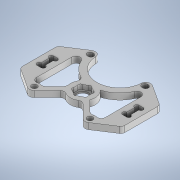
# Autodesk Inventor part: Leg_joint_roll_frame
Saved by Autodesk Inventor 2020 (Build 240168000, 168)
## iProperties
Created: 2021-10-17
Part Number: Leg_joint_roll_frame
Material: アルミニウム 2014-T4
Document SubType Name: Modeling
Designer: Masato Kubotera
Density: 2.8 g/cm^3
Appearance: 滑らか - 淡い灰色
Description: A2017 T3
Mass: 6.35026 g
Surface Area: 26.3941 cm^2
Volume: 2.26795 cm^3
Author: Masato Kubotera
Autodesk Inventor part; units mm, degrees
ref_plane "YZ Plane" through (0, 0, 0) normal (1, 0, 0) x (0, 1, 0)
ref_plane "XZ Plane" through (0, 0, 0) normal (0, 1, 0) x (-1, 0, 0)
ref_plane "XY Plane" through (0, 0, 0) normal (0, 0, 1) x (1, 0, 0)
derived "Leg_joint_roll_basis.ipt"
sketch "スケッチ1" plane through (0, 0, 0) normal (0, 0, 1) x (1, 0, 0)
  line L0 (0, 47.5) -> (0, -12.4) construction
  line L1 (-12.5, 47.5) -> (12.5, 47.5) construction
  line L2 (-12.5, 42.45) -> (-5.9323, -0.8988) construction
  arc A0 (-5.9323, -0.8988) -> (5.9323, -0.8988) centre (0, 0) ccw construction
  line L3 (-5.55, 45.05) -> (-3.45, 45.05) construction
  line L4 (5.55, 45.05) -> (5.55, 42.45) construction
  line L5 (5.55, 42.45) -> (3.45, 42.45) construction
  line L6 (-5.55, 42.45) -> (-5.55, 45.05) construction
  line L7 (-5.55, 45.05) -> (5.55, 42.45) construction
  line L8 (5.55, 45.05) -> (-5.55, 42.45) construction
  line L9 (-5.5, 45) -> (5.5, 45) construction
  line L10 (5.5, 45) -> (5.5, 42.5) construction
  line L11 (5.5, 42.5) -> (-5.5, 42.5) construction
  line L12 (-5.5, 42.5) -> (-5.5, 45) construction
  line L13 (-5.5, 45) -> (5.5, 42.5) construction
  line L14 (5.5, 45) -> (-5.5, 42.5) construction
  line L15 (-5.55, 43.75) -> (5.55, 43.75) construction
  arc A1 (-3.45, 45.05) -> (-5.55, 45.05) centre (-4.5, 45.05) ccw construction
  arc A2 (-5.55, 42.45) -> (-3.45, 42.45) centre (-4.5, 42.45) ccw construction
  line L16 (12.5, 42.45) -> (5.9323, -0.8988) construction
  arc A3 (5.55, 45.05) -> (3.45, 45.05) centre (4.5, 45.05) ccw construction
  arc A4 (3.45, 42.45) -> (5.55, 42.45) centre (4.5, 42.45) ccw construction
  line L17 (-3.45, 45.05) -> (3.45, 45.05) construction
  line L18 (-3.45, 42.45) -> (-5.55, 42.45) construction
  line L19 (3.45, 42.45) -> (-3.45, 42.45) construction
  line L20 (3.45, 45.05) -> (5.55, 45.05) construction
  circle A5 centre (0, 0) radius 4.05 construction
  line L21 (-13.5, 17) -> (13.5, 17) construction
  line L22 (13.5, 17) -> (13.5, -10) construction
  line L23 (13.5, -10) -> (-13.5, -10) construction
  line L24 (-13.5, -10) -> (-13.5, 17) construction
  line L25 (-13.5, 17) -> (13.5, -10) construction
  line L26 (13.5, 17) -> (-13.5, -10) construction
  arc A6 (-13.5, 18.35) -> (-13.5, 15.65) centre (-13.5, 17) ccw projected
  circle A7 centre (-13.5, -10) radius 1.35 projected
  line L27 (-24.81, 12.5) -> (-24.81, -5.5) projected
  circle A8 centre (-13.5, -10) radius 2.4 construction
  line L28 (-24.81, -5.5) -> (-14.2125, -12.4) projected
  line L29 (-21.75, 7.5) -> (-19.75, 7.5) construction
  line L30 (-19.75, 7.5) -> (-19.75, -0.5) construction
  line L31 (-19.75, -0.5) -> (-21.75, -0.5) construction
  line L32 (-21.75, -0.5) -> (-21.75, 7.5) construction
  line L33 (-21.75, 7.5) -> (-19.75, -0.5) construction
  line L34 (-19.75, 7.5) -> (-21.75, -0.5) construction
  line L35 (-21.76, 7.51) -> (-19.74, 7.51) projected
  line L36 (-19.74, 7.51) -> (-19.74, 5.41) construction
  line L37 (-19.74, -0.51) -> (-21.76, -0.51) projected
  line L38 (-21.76, -0.51) -> (-21.76, 1.59) construction
  line L39 (-21.76, 7.51) -> (-19.74, -0.51) construction
  line L40 (-19.74, 7.51) -> (-21.76, -0.51) construction
  arc A9 (-21.76, 7.51) -> (-21.76, 5.41) centre (-21.76, 6.46) ccw projected
  line L41 (-20.75, 7.51) -> (-20.75, -0.51) construction
  line L42 (-21.76, 3.5) -> (-19.74, 3.5) construction
  arc A10 (-19.74, 5.41) -> (-19.74, 7.51) centre (-19.74, 6.46) ccw projected
  arc A11 (-21.76, 1.59) -> (-21.76, -0.51) centre (-21.76, 0.54) ccw projected
  arc A12 (-19.74, -0.51) -> (-19.74, 1.59) centre (-19.74, 0.54) ccw projected
  line L43 (-24.81, 12.5) -> (-14.2125, 19.4) projected
  line L44 (-13.5, 18.35) -> (-13, 18.35) projected
  line L45 (-13.5, 15.65) -> (-13, 15.65) projected
  arc A13 (-13, 15.65) -> (-13, 18.35) centre (-13, 17) ccw projected
  line L46 (-21.76, 5.41) -> (-21.76, 7.51) construction
  line L47 (-21.76, 1.59) -> (-21.76, 5.41) projected
  line L48 (-19.74, 1.59) -> (-19.74, -0.51) construction
  line L49 (-19.74, 5.41) -> (-19.74, 1.59) projected
  line L50 (19.74, 5.41) -> (19.74, 1.59) projected
  line L51 (21.76, 1.59) -> (21.76, 5.41) projected
  arc A14 (21.76, 5.41) -> (21.76, 7.51) centre (21.76, 6.46) ccw projected
  line L52 (21.76, 7.51) -> (19.74, 7.51) projected
  arc A15 (19.74, 7.51) -> (19.74, 5.41) centre (19.74, 6.46) ccw projected
  arc A16 (21.76, -0.51) -> (21.76, 1.59) centre (21.76, 0.54) ccw projected
  line L53 (19.74, -0.51) -> (21.76, -0.51) projected
  arc A17 (19.74, 1.59) -> (19.74, -0.51) centre (19.74, 0.54) ccw projected
  line L54 (24.81, 12.5) -> (24.81, -5.5) projected
  line L55 (24.81, 12.5) -> (14.2125, 19.4) projected
  arc A18 (13, 18.35) -> (13, 15.65) centre (13, 17) ccw projected
  line L56 (13.5, 18.35) -> (13, 18.35) projected
  arc A19 (13.5, 15.65) -> (13.5, 18.35) centre (13.5, 17) ccw projected
  line L57 (24.81, -5.5) -> (14.2125, -12.4) projected
  circle A20 centre (13.5, -10) radius 1.35 projected
  line L58 (13.5, 15.65) -> (13, 15.65) projected
  line L59 (-14.2125, -12.4) -> (14.2125, -12.4) projected
  line L60 (-14.2125, 19.4) -> (-11.0486, 19.4) projected
  circle A21 centre (0, 18) radius 5.05 construction
  circle A22 centre (-13.5, 17) radius 2.4 construction
  arc A23 (-11.0486, 19.4) -> (11.0486, 19.4) centre (0, 18) ccw projected
  line L61 (11.0486, 19.4) -> (14.2125, 19.4) projected
  circle A24 centre (0, 26.5) radius 1.35 construction
  circle A25 centre (-8.5, 18) radius 1.35 construction
  circle A26 centre (0, 9.5) radius 1.35 construction
  circle A27 centre (8.5, 18) radius 1.35 construction
  arc A28 (5.713, 37.8333) -> (-5.713, 37.8333) centre (0, 36) ccw construction
  circle A29 centre (0, 36) radius 2.25 construction
  circle A30 centre (0, 0) radius 2.75 projected
  circle A31 centre (0, 0) radius 2.1 construction
  line L62 (0, -4.053) -> (-0.9093, -3.528) construction
  line L63 (-3.51, -2.0265) -> (-3.51, -0.9765) construction
  line L64 (-3.51, 2.0265) -> (-2.6007, 2.5515) construction
  line L65 (0, 4.053) -> (3.51, 2.0265) projected
  line L66 (3.51, 2.0265) -> (3.51, 0.9765) construction
  line L67 (3.51, -2.0265) -> (2.6007, -2.5515) construction
  arc A32 (0.9093, 3.528) -> (-0.9093, 3.528) centre (0, 3.003) ccw projected
  arc A33 (-2.6007, 2.5515) -> (-3.51, 0.9765) centre (-2.6007, 1.5015) ccw projected
  arc A34 (-3.51, -0.9765) -> (-2.6007, -2.5515) centre (-2.6007, -1.5015) ccw projected
  arc A35 (-0.9093, -3.528) -> (0.9093, -3.528) centre (0, -3.003) ccw projected
  arc A36 (2.6007, -2.5515) -> (3.51, -0.9765) centre (2.6007, -1.5015) ccw projected
  arc A37 (3.51, 0.9765) -> (2.6007, 2.5515) centre (2.6007, 1.5015) ccw projected
  line L68 (-0.9093, 3.528) -> (0, 4.053) construction
  line L69 (-2.6007, 2.5515) -> (-0.9093, 3.528) projected
  line L70 (-3.51, 0.9765) -> (-3.51, 2.0265) construction
  line L71 (-3.51, -0.9765) -> (-3.51, 0.9765) projected
  line L72 (-2.6007, -2.5515) -> (-3.51, -2.0265) construction
  line L73 (-0.9093, -3.528) -> (-2.6007, -2.5515) projected
  line L74 (0.9093, -3.528) -> (0, -4.053) construction
  line L75 (2.6007, -2.5515) -> (0.9093, -3.528) projected
  line L76 (3.51, -0.9765) -> (3.51, -2.0265) construction
  line L77 (3.51, 0.9765) -> (3.51, -0.9765) projected
  circle A38 centre (0, 0) radius 3 construction
  line L78 (-16.75, 14.168) -> (-16.75, -7.168)
  line L79 (-16.75, 14.168) -> (-15.12, 15.2292)
  arc A39 (-15.12, 15.2292) -> (-13.7246, 14.6105) centre (-13.5, 17) ccw
  line L80 (-16.75, -7.168) -> (-15.12, -8.2292)
  arc A40 (-4.0263, 4.4485) -> (-5.6149, -2.1149) centre (0, 0) ccw
  arc A41 (-13.7246, 14.6105) -> (-4.0263, 4.4485) centre (0, 18) ccw
  line L81 (-5.6149, -2.1149) -> (-11.8029, -8.3029)
  arc A42 (-11.8029, -8.3029) -> (-15.12, -8.2292) centre (-13.5, -10) ccw
  line L82 (16.75, 14.168) -> (16.75, -7.168)
  line L83 (16.75, 14.168) -> (15.12, 15.2292)
  arc A43 (13.7246, 14.6105) -> (15.12, 15.2292) centre (13.5, 17) ccw
  line L84 (16.75, -7.168) -> (15.12, -8.2292)
  arc A44 (5.6149, -2.1149) -> (4.0263, 4.4485) centre (0, 0) ccw
  arc A45 (4.0263, 4.4485) -> (13.7246, 14.6105) centre (0, 18) ccw
  line L85 (5.6149, -2.1149) -> (11.8029, -8.3029)
  arc A46 (15.12, -8.2292) -> (11.8029, -8.3029) centre (13.5, -10) ccw
  circle A47 centre (-9.5, 45) radius 1.6 projected
  circle A48 centre (9.5, 45) radius 1.6 projected
  line L86 (-12.5, 42.45) -> (-12.5, 47.5) projected
  line L87 (12.5, 47.5) -> (12.5, 42.45) projected
  arc A49 (-8.4171, 15.5014) -> (-9.1609, 20.4111) centre (-8.5, 18) ccw projected
  arc A50 (9.1609, 20.4111) -> (8.4171, 15.5014) centre (8.5, 18) ccw projected
  circle A51 centre (0, 9.5) radius 2.5 projected
  circle A52 centre (0, 18) radius 10.55 construction
  circle A53 centre (0, 18) radius 11.5 projected
  line L88 (-10.95, 21.5139) -> (-5.713, 37.8333) projected
  line L89 (5.713, 37.8333) -> (10.95, 21.5139) projected
  arc A54 (-4.2953, -4.1894) -> (4.2953, -4.1894) centre (0, 0) ccw
  arc A55 (-14.8095, -12.0113) -> (-11.8029, -11.6971) centre (-13.5, -10) ccw
  line L90 (-11.8029, -11.6971) -> (-4.2953, -4.1894)
  arc A56 (11.8029, -11.6971) -> (14.8095, -12.0113) centre (13.5, -10) ccw
  line L91 (11.8029, -11.6971) -> (4.2953, -4.1894)
  line L92 (2.0265, 32.49) -> (0.9765, 32.49) construction
  line L93 (-2.0265, 32.49) -> (-2.5515, 33.3993) construction
  line L94 (-4.053, 36) -> (-3.528, 36.9093) construction
  line L95 (-2.0265, 39.51) -> (-0.9765, 39.51) construction
  line L96 (2.0265, 39.51) -> (2.5515, 38.6007) construction
  line L97 (4.053, 36) -> (3.528, 35.0907) projected
  arc A57 (-0.9765, 39.51) -> (-2.5515, 38.6007) centre (-1.5015, 38.6007) ccw projected
  arc A58 (-3.528, 36.9093) -> (-3.528, 35.0907) centre (-3.003, 36) ccw projected
  arc A59 (-2.5515, 33.3993) -> (-0.9765, 32.49) centre (-1.5015, 33.3993) ccw projected
  arc A60 (0.9765, 32.49) -> (2.5515, 33.3993) centre (1.5015, 33.3993) ccw projected
  arc A61 (3.528, 35.0907) -> (3.528, 36.9093) centre (3.003, 36) ccw projected
  arc A62 (2.5515, 38.6007) -> (0.9765, 39.51) centre (1.5015, 38.6007) ccw projected
  line L98 (-2.5515, 38.6007) -> (-2.0265, 39.51) construction
  line L99 (-3.528, 36.9093) -> (-2.5515, 38.6007) projected
  line L100 (-3.528, 35.0907) -> (-4.053, 36) construction
  line L101 (-2.5515, 33.3993) -> (-3.528, 35.0907) projected
  line L102 (-0.9765, 32.49) -> (-2.0265, 32.49) construction
  line L103 (0.9765, 32.49) -> (-0.9765, 32.49) projected
  line L104 (2.5515, 33.3993) -> (2.0265, 32.49) construction
  line L105 (3.528, 35.0907) -> (2.5515, 33.3993) projected
  line L106 (3.528, 36.9093) -> (4.053, 36) construction
  line L107 (2.5515, 38.6007) -> (3.528, 36.9093) projected
  line L108 (-0.9765, 39.51) -> (0.9765, 39.51) projected
  line L109 (0.9765, 39.51) -> (2.0265, 39.51) construction
  circle A63 centre (0, 0) radius 6 projected
  point P0 (0, 43.75)
  point P1 (0, 3.5)
  point P2 (-20.75, 3.5)
  point P3 (-24.81, 3.5)
  point P4 (-13.5, 3.5)
  point P5 (2.6007, 2.5515)
  point P6 (-12.5059, -12.4)
  point P7 (14.8095, -12.0113)
  point P8 (11.4145, 19.4)
  point P9 (12.5471, 18.2717)
  point P10 (12.3579, 15.8125)
  point P11 (-12.3579, 15.8125)
  point P12 (-12.5471, 18.2717)
  point P13 (-11.4145, 19.4)
  point P14 (-11.8029, -11.6971)
  point P15 (-4.0263, 4.4485)
  point P16 (4.0263, 4.4485)
  point P17 (4.2953, -4.1894)
  point P18 (-4.2953, -4.1894)
  point P19 (-5.6149, -2.1149)
  point P20 (-5.6149, -2.1149)
  point P21 (-4.2953, -4.1894)
  point P22 (4.2953, -4.1894)
  point P23 (4.0263, 4.4485)
  point P24 (-4.0263, 4.4485)
  dimension "d1" = 3
  dimension "d2" = 3
  dimension "d4" = 3
  dimension "d5" = 6
  constraints: 29 point on circle, 20 end point, 15 horizontal alignment, 11 centre point, 4 coincident, 3 concentric, 3 equal radius, 2 parallel, 2 point on line, 2 symmetric about line, 1 collinear, 1 tangent, 6 other
  measures "d1" distance between parallel lines of L43 L79
  measures "d2" distance between parallel lines of L78 L30
  measures "d4" radial gap between concentric circles of A41 A23
  measures "d5" radius of A40
extrude "押し出し1" add sketch "スケッチ1" along normal blind 3 contours L43 L60 A53 L61 L55 L54 L57 A56 L91 A63 L85 A46 L84 L82 L83 A43 A45 A41 A39 L79 L78 L80 A42 L81 L90 A55 L28 L27 | L60 A23 L61 A53 | A63 A40 A44 A54 picked at (10.8928, 15.38)
extrude "押し出し2" add sketch "スケッチ1" along normal blind 0.8 contours A32 L65 | L65 A37 L77 A36 L75 A35 L73 A34 L71 A33 L69 A32 | A37 L65
fillet "フィレット1" radius 2 10 edges at (14.2125, 19.4, 1.5) (11.0486, 19.4, 1.5) (24.81, 12.5, 1.5) (24.81, -5.5, 1.5) (-24.81, -5.5, 1.5) (-24.81, 12.5, 1.5) (-14.2125, 19.4, 1.5) (-11.0486, 19.4, 1.5) (-4.2953, -4.1894, 1.5) (4.2953, -4.1894, 1.5)
fillet "フィレット2" radius 2 14 edges at (-13.7246, 14.6105, 1.5) (-15.12, 15.2292, 1.5) (-16.75, 14.168, 1.5) (-4.0263, 4.4485, 1.5) (-5.6149, -2.1149, 1.5) (-11.8029, -8.3029, 1.5) (-15.12, -8.2292, 1.5) (-16.75, -7.168, 1.5) (13.7246, 14.6105, 1.5) (15.12, 15.2292, 1.5) (16.75, 14.168, 1.5) (16.75, -7.168, 1.5) (15.12, -8.2292, 1.5) (11.8029, -8.3029, 1.5)
equation "\"d2\" = d1"
equation "\"d4\" = d1"
equation "\"d3\" = d1"
